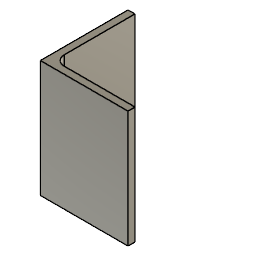
L-75×75×6 (Autodesk Fusion 360 design; units mm, degrees)
Autodesk Fusion 360 part; units mm, degrees
note: some values were not read from the file. Set by a fixed rule: which sketch regions a step uses.
sketch "スケッチ1" plane through (0, 0, 0) normal (0, 0, 1) x (1, 0, 0)
  line L0 (0, 75) -> (0, 0)
  line L1 (6, 14.5) -> (6, 75)
  line L2 (75, 6) -> (14.5, 6)
  line L3 (0, 0) -> (75, 0)
  arc A0 (6, 14.5) -> (14.5, 6) centre (14.5, 14.5) ccw
  line L4 (75, 0) -> (75, 6)
  line L5 (6, 75) -> (0, 75)
extrude "押し出し1" add sketch "スケッチ1" along normal blind 100
